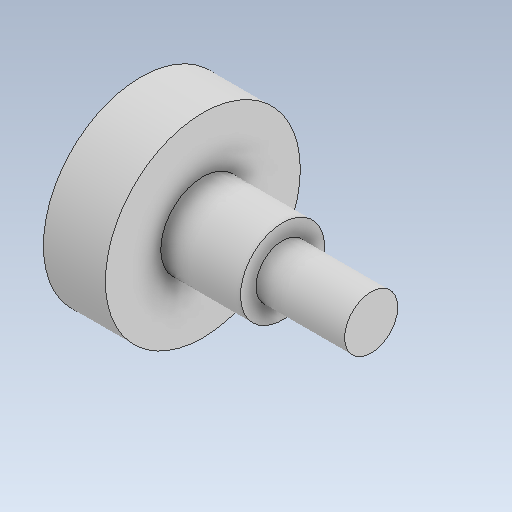
# Autodesk Inventor part: guia
Saved by Autodesk Inventor 2020 (Build 240168000, 168)
## iProperties
Created: 2021-03-26
Part Number: guia
Material: Generic
Document SubType Name: Modeling
Designer: super
Density: 1 g/cm^3
Appearance: Default
Author: super
Autodesk Inventor part; units mm, degrees
ref_plane "YZ Plane" through (0, 0, 0) normal (1, 0, 0) x (0, 1, 0)
ref_plane "XZ Plane" through (0, 0, 0) normal (0, 1, 0) x (-1, 0, 0)
ref_plane "XY Plane" through (0, 0, 0) normal (0, 0, 1) x (1, 0, 0)
sketch "Sketch1" plane through (0, 0, 0) normal (0, 0, 1) x (1, 0, 0)
  line L0 (-1.633, 4.75) -> (-10.633, 4.75)
  line L1 (-10.633, 4.75) -> (-10.633, 11)
  line L2 (-10.633, 11) -> (-17.633, 11)
  line L3 (-17.633, 11) -> (-17.633, 0)
  line L4 (-17.633, 0) -> (8.367, 0)
  line L5 (-1.633, 4.75) -> (-1.633, 3)
  line L6 (-1.633, 3) -> (8.367, 3)
  line L7 (8.367, 3) -> (8.367, 0)
  point P0 (0, 0)
  dimension "d3" = 9
  dimension "d5" = 11
  dimension "d6" = 7
  dimension "d7" = 1.75
  dimension "d8" = 3
  dimension "d9" = 4.75
  constraints: 16 end point, 4 perpendicular, 2 vertical, 1 horizontal
  measures "d3" distance of L0.start L0.end
  measures "d5" distance of L2.end L3.end
  measures "d6" distance of L1.end L2.end
  measures "d7" distance of L0.start L5.end
  measures "d8" distance of L6.end L4.end
  measures "d9" vertical distance of L4.end L0.start
revolve "Revolution1" add sketch "Sketch1" angle 360 about axis through (-17.633, 0, 0) along (1, 0, 0)
body "Solid1"
